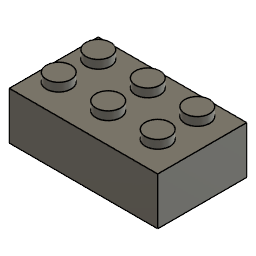
self_study_lego_block (Autodesk Fusion 360 design; units mm, degrees)
part number: 2026-07-06-14-18-54-309
Autodesk Fusion 360 part; units mm, degrees
sketch "Sketch1" plane through (0, 0, 0) normal (0, 1, 0) x (1, 0, 0)
  line L0 (0, 0) -> (30, 0)
  line L1 (30, 0) -> (30, -18)
  line L2 (30, -18) -> (0, -18)
  line L3 (0, -18) -> (0, 0)
  dimension "d1" = 30
  dimension "d2" = 18
  constraint horizontal L0
  constraint vertical L1
  constraint horizontal L2
  constraint vertical L3
  constraint coincident L0.start L3.end
  measures "d1" distance of L0.start L0.end
  measures "d2" distance of L0.start L2.end
extrude "Extrude1" add sketch "Sketch1" along normal blind 9.6
sketch "Sketch2" plane through (0, 9.6, 0) normal (0, 1, 0) x (-1, 0, 0)
  line L0 (0, 18) -> (-30, 18)
  line L1 (-30, 18) -> (-30, 0)
  line L2 (-30, 0) -> (0, 0)
  line L3 (0, 0) -> (0, 18)
  circle A0 centre (-3.9, 3.9) radius 2.5
  dimension "d5" = 5
  dimension "d6" = 3.9
  dimension "d7" = 3.9
  measures "d5" diameter of A0
  measures "d6" distance of L2 A0.centre
  measures "d7" distance of L3 A0.centre
extrude "Extrude2" add sketch "Sketch2" along normal blind 1.7 contours A0
pattern_linear "R-Pattern1" count 3 spacing 10 along (1, 0, 0) count 2 spacing 8 along (0, 0, 1) of "Extrude2"
shell "Shell1" thickness 1.5 removed faces 1 at (10, 0, 6)
